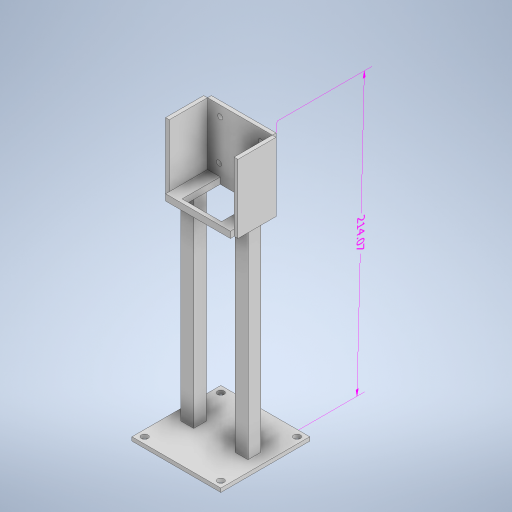
# Autodesk Inventor part: depth-camera-base
Saved by Autodesk Inventor 2023 (Build 270158000, 158)
## iProperties
Created: 2024-04-08
Part Number: depth-camera-base
Material: Genérico
Document SubType Name: Modeling
Designer: inigo
Density: 1 g/cm^3
Appearance: Valor por defecto
Author: inigo
Autodesk Inventor part; units mm, degrees
ref_plane "YZ Plane" through (0, 0, 0) normal (1, 0, 0) x (0, 1, 0)
ref_plane "XZ Plane" through (0, 0, 0) normal (0, 1, 0) x (-1, 0, 0)
ref_plane "XY Plane" through (0, 0, 0) normal (0, 0, 1) x (1, 0, 0)
sketch "Boceto1" plane through (0, 0, 0) normal (0, 1, 0) x (-1, 0, 0)
  line L0 (25.5, 15) -> (-25.5, 15)
  line L1 (-25.5, 15) -> (-25.5, -15)
  line L2 (-25.5, -15) -> (25.5, -15)
  line L3 (25.5, -15) -> (25.5, 15)
  line L4 (25.5, 15) -> (-25.5, -15) construction
  line L5 (-25.5, 15) -> (25.5, -15) construction
  line L6 (-15.5, 15) -> (-15.5, -15)
  line L7 (0, 15) -> (0, 11.847)
  line L8 (-25.5, 0) -> (-22.3332, 0)
  line L9 (25.5, 15) -> (25.5, -15)
  line L10 (15.5, 15) -> (15.5, -15)
  line L11 (25.5, 0) -> (22.3332, 0)
  line L12 (-25.5, -15) -> (-25.5, 15)
  line L13 (-25.5, 0) -> (-22.3332, 0)
  line L14 (-25.5, 15) -> (-25.5, -15)
  point P0 (0, 0)
  point P1 (31.5, 22.5)
  dimension "d2" = 10
  dimension "d21" = 51
  dimension "d22" = 30
  constraints: 30 end point, 5 symmetric about line, 4 midpoint, 2 horizontal, 2 parallel, 2 perpendicular, 2 point on line, 1 vertical
  measures "d2" distance between parallel lines of L6 L1
  measures "d21" distance between parallel lines of L3 L1
  measures "d22" distance between parallel lines of L0 L2
extrude "Extrusión1" add sketch "Boceto1" along normal blind 5 contours L3 L2 L10 L0 | L6 L2 L1 L0
sketch "Boceto4" plane through (0, 0, 0) normal (0, 1, 0) x (-1, 0, 0)
  line L0 (-28.5, 18) -> (28.5, 18)
  line L1 (28.5, 18) -> (28.5, -18)
  line L2 (28.5, -18) -> (-28.5, -18)
  line L3 (-28.5, -18) -> (-28.5, 18)
  line L4 (-28.5, 18) -> (28.5, -18) construction
  line L5 (28.5, 18) -> (-28.5, -18) construction
  line L6 (28.5, -15) -> (-28.5, -15)
  line L7 (-28.5, 15) -> (28.5, 15)
  line L8 (25.5, -18) -> (25.5, 18)
  line L9 (-25.5, 18) -> (-25.5, -18)
  line L10 (-25.5, -15) -> (-15.5, -15) projected
  point P0 (0, 0)
  point P1 (-25.5, -15)
  point P2 (-25.5, 15)
  point P3 (25.5, 15)
  point P4 (25.5, -15)
  dimension "d23" = 57
  dimension "d24" = 36
  dimension "d27" = 0
  constraints: 20 end point, 8 point on line, 5 perpendicular, 2 midpoint, 2 parallel, 1 horizontal
  measures "d23" distance of L1.end L2.end
  measures "d24" distance of L0.end L1.end
  measures "d27" distance between parallel lines of L6 L10
extrude "Extrusión4" add sketch "Boceto4" along normal blind 5 contours L0 L8 L7 L9 | L7 L9 L6 L3 | L7 L1 L6 L8 | L6 L8 L2 L9
sketch "Boceto5" plane through (0, 5, 0) normal (0, 1, 0) x (1, 0, 0)
  line L0 (25.5, 18) -> (-25.5, 18) projected
  line L1 (25.5, 15) -> (25.5, 18) projected
  line L2 (-25.5, 18) -> (25.5, 18)
  line L3 (25.5, 18) -> (25.5, 15)
  line L4 (25.5, 15) -> (-25.5, 15)
  line L5 (-25.5, 15) -> (-25.5, 18)
  point P0 (0, 0)
  constraints: 8 end point, 2 parallel, 1 horizontal, 1 perpendicular
extrude "Extrusión5" add sketch "Boceto5" along normal blind 49
sketch "Boceto6" plane through (-15.5, 0, -15) normal (0, 0, 1) x (1, 0, 0)
  circle A0 centre (32, 45) radius 2
  line L0 (41, 5) -> (41, 54) projected
  line L1 (-10, 54) -> (41, 54) projected
  line L2 (-10, 5) -> (-10, 54) projected
  line L3 (-10, 29.5) -> (15.5, 29.5)
  line L4 (15.5, 29.5) -> (15.5, 54)
  circle A1 centre (0, 46) radius 2
  circle A2 centre (-1, 14) radius 2
  circle A3 centre (31, 13) radius 2
  point P0 (15.5, 0)
  dimension "d30" = 4
  dimension "d31" = 9
  dimension "d32" = 9
  dimension "d35" = 360
  constraints: 4 centre point, 4 end point, 2 midpoint, 1 coincident, 1 horizontal, 9 other
  measures "d30" diameter of A0
  measures "d31" distance from line of L0 A0.centre
  measures "d32" distance from line of L1 A0.centre
extrude "Extrusión6" cut sketch "Boceto6" against normal blind 49 contours A0 | A1 | A2 | A3
sketch "Boceto7" plane through (0, 5, 0) normal (0, 1, 0) x (1, 0, 0)
  line L0 (-28.5, 15) -> (-28.5, -15) projected
  line L1 (-28.5, 15) -> (-25.5, 15)
  line L2 (-25.5, 15) -> (-25.5, -15)
  line L3 (-25.5, -15) -> (-28.5, -15)
  line L4 (-28.5, -15) -> (-28.5, 15)
  line L5 (28.5, 15) -> (25.5, 15) projected
  line L6 (25.5, -15) -> (28.5, -15) projected
  line L7 (28.5, 15) -> (25.5, 15)
  line L8 (25.5, 15) -> (25.5, -15)
  line L9 (25.5, -15) -> (28.5, -15)
  line L10 (28.5, -15) -> (28.5, 15)
  point P0 (0, 0)
  point P1 (25.5, -18)
  constraints: 16 end point, 4 parallel, 2 horizontal, 2 perpendicular
extrude "Extrusión7" add sketch "Boceto7" along normal blind 49
sketch "Boceto9" plane through (0, 0, 0) normal (0, -1, 0) x (1, 0, 0)
  line L0 (-15.5, 15) -> (-15.5, -15) projected
  line L1 (-25.5, 15) -> (-15.5, 15)
  line L2 (-15.5, 0) -> (-28.5, 0)
  line L3 (-28.5, -15) -> (-28.5, 15) projected
  line L4 (-26.3951, 5) -> (-16.3951, 5)
  line L5 (-16.3951, 5) -> (-16.3951, -5)
  line L6 (-16.3951, -5) -> (-26.3951, -5)
  line L7 (-26.3951, -5) -> (-26.3951, 5)
  line L8 (-26.3951, 5) -> (-16.3951, -5) construction
  line L9 (-16.3951, 5) -> (-26.3951, -5) construction
  line L10 (26.3951, -5) -> (16.3951, -5)
  line L11 (16.3951, -5) -> (16.3951, 5)
  line L12 (16.3951, 5) -> (26.3951, 5)
  line L13 (26.3951, 5) -> (26.3951, -5)
  line L14 (26.3951, -5) -> (16.3951, 5) construction
  line L15 (16.3951, -5) -> (26.3951, 5) construction
  point P0 (0, 0)
  point P1 (-21.3951, 0)
  point P2 (21.3951, 0)
  dimension "d41" = 10
  dimension "d42" = 10
  dimension "d45" = 360
  constraints: 28 end point, 4 midpoint, 2 horizontal, 2 parallel, 1 perpendicular, 1 point on line, 23 other
  measures "d41" distance of L5.end L6.end
  measures "d42" distance of L4.end L5.end
extrude "Extrusión8" add sketch "Boceto9" along normal blind 160
sketch "Boceto11" plane through (0, -160, 0) normal (0, -1, 0) x (1, 0, 0)
  line L0 (-35, 35) -> (35, 35)
  line L1 (35, 35) -> (35, -35)
  line L2 (35, -35) -> (-35, -35)
  line L3 (-35, -35) -> (-35, 35)
  line L4 (-35, 35) -> (35, -35) construction
  line L5 (35, 35) -> (-35, -35) construction
  line L6 (-35, -35) -> (35, -35)
  line L7 (35, -35) -> (35, 35)
  line L8 (35, 35) -> (-35, 35)
  line L9 (-35, 35) -> (-35, -35)
  line L10 (-35, -35) -> (35, 35) construction
  line L11 (35, -35) -> (-35, 35) construction
  line L12 (30, 30) -> (-30, 30)
  line L13 (-30, 30) -> (-30, -30)
  line L14 (-30, -30) -> (30, -30)
  line L15 (30, -30) -> (30, 30)
  line L16 (30, 30) -> (-30, -30) construction
  line L17 (-30, 30) -> (30, -30) construction
  circle A0 centre (-30, 30) radius 2.6
  circle A1 centre (30, 30) radius 2.6
  circle A2 centre (30, -30) radius 2.6
  circle A3 centre (-30, -30) radius 2.6
  line L18 (-26.3951, 5) -> (-16.3951, 5) projected
  line L19 (-16.3951, 5) -> (-16.3951, -5) projected
  line L20 (-26.3951, 5) -> (-16.3951, 5)
  line L21 (-16.3951, 5) -> (-16.3951, -5)
  line L22 (-16.3951, -5) -> (-26.3951, -5)
  line L23 (-26.3951, -5) -> (-26.3951, 5)
  line L24 (16.3951, 5) -> (26.3951, 5) projected
  line L25 (26.3951, 5) -> (26.3951, -5) projected
  line L26 (16.3951, 5) -> (26.3951, 5)
  line L27 (26.3951, 5) -> (26.3951, -5)
  line L28 (26.3951, -5) -> (16.3951, -5)
  line L29 (16.3951, -5) -> (16.3951, 5)
  point P0 (0, 0)
  point P1 (0, 0)
  dimension "d52" = 70
  dimension "d53" = 70
  dimension "d54" = 70
  dimension "d55" = 70
  dimension "d56" = 60
  dimension "d57" = 5.2
  dimension "d58" = 5.2
  dimension "d59" = 5.2
  dimension "d60" = 5.2
  constraints: 52 end point, 10 parallel, 6 midpoint, 5 horizontal, 5 perpendicular, 4 centre point, 4 coincident, 1 point on line
  measures "d52" distance of L1.end L2.end
  measures "d53" distance of L0.end L1.end
  measures "d54" distance of L8.end L8.start
  measures "d55" distance of L8.start L7.start
  measures "d56" distance of L13.end L12.end
  measures "d57" diameter of A0
  measures "d58" diameter of A1
  measures "d59" diameter of A2
  measures "d60" diameter of A3
extrude "Extrusión9" add sketch "Boceto11" against normal blind 3 contours L0 L1 L2 L3 | L12 A1 L15 A2 L14 A3 L13 A0
